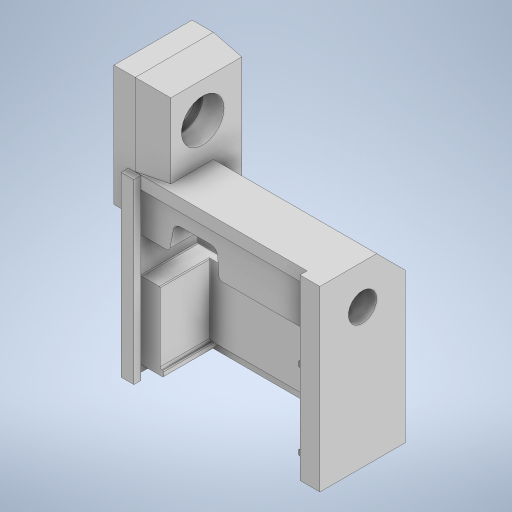
# Autodesk Inventor part: LimitSwitch Container
Saved by Autodesk Inventor 2023 (Build 270158000, 158)
## iProperties
Created: 2019-04-18
Part Number: LimitSwitch Container
Material: Generic
Document SubType Name: Modeling
Designer: Parker
Density: 1 g/cm^3
Appearance: Default
Author: Parker
Autodesk Inventor part; units mm, degrees
ref_plane "YZ Plane" through (0, 0, 0) normal (1, 0, 0) x (0, 1, 0)
sketch "Sketch1" plane through (0, 0, 0) normal (0, 0, 1) x (1, 0, 0)
  line L0 (-11.5, -20) -> (11.5, -20)
  line L1 (13.5, -18) -> (13.5, 18)
  line L2 (11.5, 20) -> (-11.5, 20)
  line L3 (-13.5, 18) -> (-13.5, -18)
  line L4 (-13.5, -20) -> (13.5, 20) construction
  line L5 (13.5, -20) -> (-13.5, 20) construction
  arc A0 (13.5, 18) -> (11.5, 20) centre (11.5, 18) ccw
  arc A1 (-11.5, 20) -> (-13.5, 18) centre (-11.5, 18) ccw
  arc A2 (-13.5, -18) -> (-11.5, -20) centre (-11.5, -18) ccw
  arc A3 (11.5, -20) -> (13.5, -18) centre (11.5, -18) ccw
  line L6 (12.7, 18) -> (12.7, -18)
  arc A4 (11.5, -19.2) -> (12.7, -18) centre (11.5, -18) ccw
  line L7 (11.5, -19.2) -> (-11.5, -19.2)
  arc A5 (-12.7, -18) -> (-11.5, -19.2) centre (-11.5, -18) ccw
  line L8 (-12.7, -18) -> (-12.7, 18)
  arc A6 (-11.5, 19.2) -> (-12.7, 18) centre (-11.5, 18) ccw
  line L9 (-11.5, 19.2) -> (11.5, 19.2)
  arc A7 (12.7, 18) -> (11.5, 19.2) centre (11.5, 18) ccw
  point P0 (0, 0)
  dimension "d0" = 27
  dimension "d1" = 40
  dimension "d2" = 2
  dimension "d3" = 0.8
  constraints: 20 end point, 16 point on circle, 8 centre point, 8 point on line, 8 tangent, 4 parallel, 3 equal radius, 2 midpoint, 2 perpendicular, 1 horizontal, 7 other
  measures "d0" distance of L4.end L5.end
  measures "d1" distance of L5.start L4.end
  measures "d2" radius of A0
  measures "d3" distance between parallel lines of L1 L6
extrude "Extrusion1" add sketch "Sketch1" along normal blind 10
sketch "Sketch2" plane through (13.5, -18, 0) normal (1, 0, 0) x (0, 0, -1)
  line L0 (-10, 0) -> (-10, 36) projected
  line L1 (0, 38) -> (-10, 38) projected
  point P0 (0, 18)
  point P1 (-5, 33.5)
  dimension "d6" = 5
  dimension "d7" = 4.5
  measures "d6" distance from line of L0 point (-5, 33.5)
  measures "d7" distance from line of L1 point (-5, 33.5)
ref_plane "Work Plane1" through (0, 0, 9) normal (0, 0, 1) x (1, 0, 0)
sketch "Sketch3" plane through (0, 0, 9) normal (0, 0, 1) x (1, 0, 0)
  arc A0 (-13.5, -18) -> (-11.5, -20) centre (-11.5, -18) ccw projected
  line L0 (-11.5, -20) -> (11.5, -20) projected
  arc A1 (11.5, -20) -> (13.5, -18) centre (11.5, -18) ccw projected
  line L1 (13.5, -18) -> (13.5, 18) projected
  arc A2 (13.5, 18) -> (11.5, 20) centre (11.5, 18) ccw projected
  line L2 (11.5, 20) -> (-11.5, 20) projected
  arc A3 (-11.5, 20) -> (-13.5, 18) centre (-11.5, 18) ccw projected
  line L3 (-13.5, 18) -> (-13.5, -18) projected
  line L4 (11.5, -19.2) -> (-11.5, -19.2) projected
  arc A4 (-12.7, -18) -> (-11.5, -19.2) centre (-11.5, -18) ccw projected
  line L5 (-12.7, -18) -> (-12.7, 18) projected
  arc A5 (-11.5, 19.2) -> (-12.7, 18) centre (-11.5, 18) ccw projected
  line L6 (-11.5, 19.2) -> (11.5, 19.2) projected
  arc A6 (12.7, 18) -> (11.5, 19.2) centre (11.5, 18) ccw projected
  line L7 (12.7, 18) -> (12.7, -18) projected
  arc A7 (11.5, -19.2) -> (12.7, -18) centre (11.5, -18) ccw projected
  line L8 (-12.7, 12.7) -> (12.7, 12.7)
  point P0 (0, 0)
  dimension "d16" = 6.5
  constraints: 2 end point, 2 point on line, 1 perpendicular
  measures "d16" distance between parallel lines of L8 L6
extrude "Extrusion2" add sketch "Sketch3" against normal blind 8 contours L8 L5 A5 L6 A6 L7
hole "Hole2" at (13.5, 15.5, 5) direction (-1, 0, 0) diameter 4 end through all
sketch "Sketch4" plane through (0, 0, 9) normal (0, 0, 1) x (1, 0, 0)
  line L0 (12.7, 18) -> (12.7, -18) projected
  line L1 (10, -2.3) -> (12.7, -2.3)
  line L2 (12.7, -2.3) -> (12.7, 7.7)
  line L3 (12.7, 7.7) -> (10, 7.7)
  line L4 (10, 7.7) -> (10, -2.3)
  line L5 (10, -2.3) -> (12.7, 7.7) construction
  line L6 (12.7, -2.3) -> (10, 7.7) construction
  line L7 (-10, -2.3) -> (-12.7, -2.3)
  line L8 (-12.7, -2.3) -> (-12.7, 7.7)
  line L9 (-12.7, 7.7) -> (-10, 7.7)
  line L10 (-10, 7.7) -> (-10, -2.3)
  line L11 (-10, -2.3) -> (-12.7, 7.7) construction
  line L12 (-12.7, -2.3) -> (-10, 7.7) construction
  arc A0 (-13.5, -18) -> (-11.5, -20) centre (-11.5, -18) ccw projected
  line L13 (-11.5, -20) -> (11.5, -20) projected
  arc A1 (11.5, -20) -> (13.5, -18) centre (11.5, -18) ccw projected
  line L14 (13.5, -18) -> (13.5, 18) projected
  arc A2 (13.5, 18) -> (11.5, 20) centre (11.5, 18) ccw projected
  line L15 (11.5, 20) -> (-11.5, 20) projected
  arc A3 (-11.5, 20) -> (-13.5, 18) centre (-11.5, 18) ccw projected
  line L16 (-13.5, 18) -> (-13.5, -18) projected
  line L17 (11.5, -19.2) -> (-11.5, -19.2) projected
  arc A4 (-12.7, -18) -> (-11.5, -19.2) centre (-11.5, -18) ccw projected
  line L18 (-12.7, -18) -> (-12.7, 18) projected
  arc A5 (-11.5, 19.2) -> (-12.7, 18) centre (-11.5, 18) ccw projected
  line L19 (-11.5, 19.2) -> (11.5, 19.2) projected
  arc A6 (12.7, 18) -> (11.5, 19.2) centre (11.5, 18) ccw projected
  line L20 (12.7, 18) -> (12.7, -18) projected
  arc A7 (11.5, -19.2) -> (12.7, -18) centre (11.5, -18) ccw projected
  line L21 (-12.7, 12.7) -> (12.7, 12.7) projected
  point P0 (0, 0)
  point P1 (11.35, 2.7)
  point P2 (-11.35, 2.7)
  dimension "d26" = 20
  dimension "d27" = 0
  dimension "d28" = 0
  dimension "d29" = 10
  dimension "d30" = 10
  dimension "d31" = 10
  dimension "d32" = 5
  constraints: 24 end point, 4 midpoint, 4 parallel, 2 horizontal, 2 perpendicular, 1 point on line
  measures "d26" distance between parallel lines of L4 L10
  measures "d27" distance between parallel lines of L18 L8
  measures "d28" distance from line of L1.start L7
  measures "d29" distance of L3.end L1.start
  measures "d30" distance of L9.end L7.start
  measures "d31" distance from line of point (0, 0) L4
  measures "d32" distance between parallel lines of L9 L21
extrude "Extrusion3" add sketch "Sketch4" against normal blind 8 contours L0 L1 L4 L3 | L9 L10 L7 L8
sketch "Sketch5" plane through (0, 0, 0) normal (0, 0, -1) x (-1, 0, 0)
  arc A0 (11.5, -20) -> (13.5, -18) centre (11.5, -18) ccw projected
  line L0 (13.5, 18) -> (13.5, -18) projected
  arc A1 (13.5, 18) -> (11.5, 20) centre (11.5, 18) ccw projected
  line L1 (-11.5, 20) -> (11.5, 20) projected
  arc A2 (-11.5, 20) -> (-13.5, 18) centre (-11.5, 18) ccw projected
  line L2 (-13.5, -18) -> (-13.5, 18) projected
  arc A3 (-13.5, -18) -> (-11.5, -20) centre (-11.5, -18) ccw projected
  line L3 (11.5, -20) -> (-11.5, -20) projected
  line L4 (-11.5, -19.2) -> (11.5, -19.2) projected
  arc A4 (-12.7, -18) -> (-11.5, -19.2) centre (-11.5, -18) ccw projected
  line L5 (-12.7, 18) -> (-12.7, -18) projected
  arc A5 (-11.5, 19.2) -> (-12.7, 18) centre (-11.5, 18) ccw projected
  line L6 (11.5, 19.2) -> (-11.5, 19.2) projected
  arc A6 (12.7, 18) -> (11.5, 19.2) centre (11.5, 18) ccw projected
  line L7 (12.7, -18) -> (12.7, 18) projected
  arc A7 (11.5, -19.2) -> (12.7, -18) centre (11.5, -18) ccw projected
  point P0 (0, 0)
extrude "Extrusion4" add sketch "Sketch5" against normal blind 1 contours A4 L5 A5 L6 A6 L7 A7 L4
sketch "Sketch6" plane through (0, 0, 9) normal (0, 0, 1) x (1, 0, 0)
  line L0 (-12.7, 12.7) -> (12.7, 12.7) projected
  line L1 (-11.7, 12.7) -> (-10.95, 16.45)
  line L2 (-10.95, 16.45) -> (-4.95, 16.45)
  line L3 (-4.95, 16.45) -> (-4.7, 12.7)
  line L4 (-12.7, -18) -> (-12.7, 18) projected
  point P0 (0, 0)
  dimension "d38" = 3.75
  dimension "d39" = 1
  dimension "d40" = 7
  dimension "d41" = 6
  dimension "d42" = 0.75
  constraints: 6 end point, 2 point on line, 1 horizontal
  measures "d38" distance between parallel lines of L0 L2
  measures "d39" distance from line of L4 L1.start
  measures "d40" distance of L1.start L3.end
  measures "d41" distance of L1.end L2.end
  measures "d42" horizontal distance of L1.start L1.end
extrude "Extrusion5" cut sketch "Sketch6" against normal blind 8
fillet "Fillet1" radius 0.5 2 edges at (-4.7, 12.7, 5) (-11.7, 12.7, 5)
fillet "Fillet2" radius 1 4 edges at (-10.95, 16.45, 7.88) (-10.95, 16.45, 2.12) (-4.95, 16.45, 7.88) (-4.95, 16.45, 2.12)
sketch "Sketch7" plane through (0, 0, 1) normal (0, 0, 1) x (1, 0, 0)
  line L0 (-10, 7.7) -> (-10, -2.3) projected
  line L1 (-10, 7.7) -> (2.5475, 7.7)
  line L2 (10, -2.3) -> (10, 7.7) projected
  line L3 (-10, -2.3) -> (10, -2.3)
  line L4 (10, -2.3) -> (10, 2.7)
  line L5 (10, 2.7) -> (3.2452, 2.7) construction
  line L6 (3.2452, 2.7) -> (2.5475, 7.7) construction
  spline S0 degree 2 poles (10, 2.7) (3.2452, 2.7) (2.5475, 7.7) knots 1 1 1 2 2 2
  point P0 (0, 0)
  constraints: 6 end point, 2 horizontal, 1 midpoint, 3 other
extrude "Extrusion6" add sketch "Sketch7" along normal blind 1
sketch "Sketch8" plane through (0, 0, 9) normal (0, 0, 1) x (1, 0, 0)
  line L0 (12.7, 7.7) -> (12.7, -2.3) projected
  line L1 (12.7, 7.7) -> (9.5, 7.7)
  line L2 (9.5, 7.7) -> (9.5, 8.5)
  line L3 (9.5, 8.5) -> (12.7, 8.5)
  line L4 (12.7, 8.5) -> (12.7, 7.7)
  line L5 (10, -2.3) -> (12.7, -2.3) projected
  line L6 (12.7, -2.3) -> (9.5, -2.3)
  line L7 (9.5, -2.3) -> (9.5, -3.1)
  line L8 (9.5, -3.1) -> (12.7, -3.1)
  line L9 (12.7, -3.1) -> (12.7, -2.3)
  line L10 (-12.7, -2.3) -> (-10, -2.3) projected
  line L11 (-12.7, -2.3) -> (-9.5, -2.3)
  line L12 (-9.5, -2.3) -> (-9.5, -3.1)
  line L13 (-9.5, -3.1) -> (-12.7, -3.1)
  line L14 (-12.7, -3.1) -> (-12.7, -2.3)
  line L15 (-10, -2.3) -> (-10, 7.7) projected
  line L16 (10, 7.7) -> (10, -2.3) projected
  point P0 (0, 0)
  dimension "d49" = 0.8
  dimension "d50" = 0.8
  dimension "d51" = 0.8
  dimension "d52" = 0.5
  dimension "d53" = 0.5
  dimension "d54" = 0.5
  constraints: 24 end point, 6 parallel, 3 horizontal, 3 perpendicular
  measures "d49" distance of L1.end L2.end
  measures "d50" distance of L6.end L7.end
  measures "d51" distance of L11.end L12.end
  measures "d52" distance between parallel lines of L12 L15
  measures "d53" distance between parallel lines of L16 L7
  measures "d54" distance between parallel lines of L16 L2
extrude "Extrusion7" add sketch "Sketch8" against normal blind 8 contours L1 L2 L3 L4 | L9 L8 L7 L6 L5 | L10 L11 L12 L13 L14
fillet "Fillet3" radius 0.25 3 edges at (10, 7.7, 5) (10, -2.3, 5.5) (-10, -2.3, 5.5)
fillet "Fillet4" radius 0.125 11 edges at (-9.5, -2.3, 5.5) (-9.5, -3.1, 5) (9.5, -3.1, 5) (9.5, -2.3, 5.5) (9.5, 7.7, 5) (9.5, 8.5, 5) (12.7, -3.1, 5) (12.7, 8.5, 5) (-12.7, 7.7, 5) (-10, 7.7, 5.5) (-12.7, -3.1, 5)
sketch "Sketch9" plane through (-11.5, -20, 0) normal (0, -1, 0) x (1, 0, 0)
  line L0 (0, 10) -> (23, 10) projected
  line L1 (11.5, 10) -> (11.5, 0) construction
  line L2 (10, 5) -> (13, 5)
  circle A0 centre (10, 5) radius 1
  circle A1 centre (13, 5) radius 1
  line L3 (10, 6) -> (13, 6)
  line L4 (13, 4) -> (10, 4)
  point P0 (11.5, 5)
  dimension "d59" = 3
  dimension "d60" = 1.5
  dimension "d61" = 2
  dimension "d62" = 2
  constraints: 8 end point, 4 point on circle, 2 centre point, 2 coincident, 2 midpoint, 2 tangent, 1 horizontal, 1 perpendicular
  measures "d59" distance of L2.start L2.end
  measures "d60" distance of point (11.5, 5) L2.end
  measures "d61" diameter of A0
  measures "d62" diameter of A1
extrude "Extrusion8" cut sketch "Sketch9" against normal up to next
sketch "Sketch11" plane through (0, 0, 10) normal (0, 0, 1) x (1, 0, 0)
  line L0 (13.5, -18) -> (13.5, 18) projected
  line L1 (13.5, -4.0701) -> (-15.3407, -4.0701)
  line L2 (-15.3407, -4.0701) -> (-15.3407, -24.8715)
  line L3 (-15.3407, -24.8715) -> (13.5, -24.8715)
  line L4 (13.5, -24.8715) -> (13.5, -4.0701)
  point P0 (0, 0)
  point P1 (13.5, -18)
  constraints: 8 end point, 2 parallel, 1 horizontal, 1 perpendicular, 1 point on line
extrude "Extrusion10" cut sketch "Sketch11" against normal through all
sketch "Sketch12" plane through (0, 0, 10) normal (0, 0, 1) x (1, 0, 0)
  line L0 (12.7, -4.0701) -> (13.5, -4.0701) projected
  line L1 (13.5, -4.0701) -> (13.5, 18) projected
  arc A0 (13.5, 18) -> (11.5, 20) centre (11.5, 18) ccw projected
  line L2 (11.5, 20) -> (-11.5, 20) projected
  arc A1 (-11.5, 20) -> (-13.5, 18) centre (-11.5, 18) ccw projected
  line L3 (-13.5, 18) -> (-13.5, -4.0701) projected
  line L4 (-13.5, -4.0701) -> (-12.7, -4.0701) projected
  line L5 (-12.7, -4.0701) -> (-12.7, 18) projected
  arc A2 (-11.5, 19.2) -> (-12.7, 18) centre (-11.5, 18) ccw projected
  line L6 (-11.5, 19.2) -> (11.5, 19.2) projected
  arc A3 (12.7, 18) -> (11.5, 19.2) centre (11.5, 18) ccw projected
  line L7 (12.7, 18) -> (12.7, -4.0701) projected
  line L8 (11.5, 20) -> (13.5, 20)
  arc A4 (13.5, 18) -> (11.5, 20) centre (11.5, 18) ccw projected
  line L9 (13.5, 20) -> (13.5, 18)
  line L10 (-13.5, 18) -> (-13.5, -4.0701) projected
  line L11 (-13.5, 18) -> (-13.5, 20)
  line L12 (-13.5, 20) -> (-11.5, 20)
  point P0 (0, 0)
  constraints: 8 end point, 2 point on line, 1 collinear, 1 horizontal, 1 perpendicular, 1 tangent
extrude "Extrusion11" add sketch "Sketch12" against normal up to surface (10 mm away) contours A0 L8 L9 | A1 L11 L12
sketch "Sketch13" plane through (-13.5, 20, 0) normal (-1, 0, 0) x (0, 0, 1)
  line L0 (0, -24.0701) -> (10, -24.0701) projected
  line L1 (10, 0) -> (10, -24.0701) projected
  line L2 (0, -24.0701) -> (0, 0) projected
  circle A0 centre (5, -4.5) radius 2 projected
  line L3 (0, 0) -> (0, -24.0701) projected
  line L4 (0, -12.9) -> (10, -12.9)
  line L5 (10, -12.9) -> (10, 12.5)
  line L6 (10, 12.5) -> (0, 12.5)
  line L7 (0, 12.5) -> (0, -12.9)
  line L8 (-1, -13.4) -> (-20.5, -13.4) projected
  line L9 (-59, 12.5) -> (-1, 12.5) projected
  line L10 (10, 0) -> (0, 0) projected
  point P0 (0, -20)
  point P1 (0, -12.9)
  point P2 (10, -12.9)
  dimension "d73" = 0.5
  dimension "d74" = 0
  constraints: 8 end point, 2 parallel, 1 horizontal, 1 perpendicular, 1 point on line
  measures "d73" distance between parallel lines of L8 L4
  measures "d74" distance between parallel lines of L9 L6
ref_plane "Work Plane2" through (-14.5, 15.5, -59) normal (1, 0, 0) x (0, 1, 0)
extrude "Extrusion12" add sketch "Sketch13" along normal up to surface (1 mm away) contours L2 L10 L1 L4 | L7 L6 L5 L10 | A0
sketch "Sketch14" plane through (-13.5, 20, 0) normal (1, 0, 0) x (0, 0, -1)
  line L0 (-10, 0) -> (0, 0) projected
  line L1 (0, 12.5) -> (0, 0) projected
  line L2 (-10, 12.5) -> (0, 12.5) projected
  line L3 (-10, 0) -> (-10, 12.5) projected
  point P0 (0, -20)
extrude "Extrusion13" add sketch "Sketch14" along normal blind 5
move faces "Move1" translate (0, 1, 0) faces at (6.1667, 20, 3.3333)
move faces "Move2" translate (0, 0, -1) faces at (4.5, 8.01, 0)
move faces "Move3" translate (1, 0, 0) faces at (13.5, 1.7915, 4.5863)
sketch "Sketch15" plane through (-8.5, 20, 0) normal (1, 0, 0) x (0, 0, -1)
  line L0 (1, 1) -> (1, 12.5) projected
  line L1 (-10, 1) -> (1, 1) projected
  point P0 (0, -20)
  point P1 (-4.5, 6.5)
  dimension "d88" = 5.5
  dimension "d89" = 5.5
  measures "d88" distance from line of L0 point (-4.5, 6.5)
  measures "d89" distance from line of L1 point (-4.5, 6.5)
hole "Hole3" at (-8.5, 26.5, 4.5) direction (-1, 0, 0) diameter 3.6 end through all counterbore diameter 6 counterbore depth 3
chamfer "Chamfer1" distance 1 distance2 4 1 edges at (-8.5, 32.5, 4.5) measured on face at (-8.5, 32, 4.5)
chamfer "Chamfer2" distance 1 distance2 4 1 edges at (-8.5, 26.25, 10) measured on face at (-8.5, 26.25, 9.5)
sketch "Sketch16" plane through (0, 0, 10) normal (0, 0, 1) x (1, 0, 0)
  line L0 (-13.5, -4.0701) -> (-13.5, 7.1) projected
  line L1 (-13.5, -4.0701) -> (-11.7, -4.0701)
  line L2 (-11.7, -4.0701) -> (-11.7, 20.9299)
  line L3 (-11.7, 20.9299) -> (-13.5, 20.9299)
  line L4 (-13.5, 20.9299) -> (-13.5, -4.0701)
  line L5 (14.5, -4.0701) -> (-13.5, -4.0701) projected
  line L6 (-8.5, 21) -> (14.5, 21) projected
  line L7 (14.5, -4.0701) -> (11.7, -4.0701)
  line L8 (11.7, -4.0701) -> (11.7, 21)
  line L9 (11.7, 21) -> (14.5, 21)
  line L10 (14.5, 21) -> (14.5, -4.0701)
  line L11 (12.7, 18) -> (12.7, -4.0701) projected
  line L12 (-12.7, -4.0701) -> (-12.7, 18) projected
  point P0 (0, 0)
  dimension "d103" = 25
  dimension "d105" = 1
  dimension "d106" = 1
  constraints: 16 end point, 4 parallel, 2 horizontal, 2 perpendicular, 1 point on line
  measures "d103" distance of L2.end L1.end
  measures "d105" distance between parallel lines of L11 L8
  measures "d106" distance between parallel lines of L12 L2
extrude "Extrusion14" add sketch "Sketch16" along normal blind 1
sketch "Sketch17" plane through (-14.5, 7.1, 10) normal (-1, 0, 0) x (0, 0, 1)
  circle A0 centre (-5.5, 19.4) radius 1.8 projected
  line L0 (0, 25.4) -> (-11, 25.4) projected
  line L1 (-11, 25.4) -> (-11, 0) projected
  line L2 (-11, 0) -> (0, 0) projected
  line L3 (0, 0) -> (0, 25.4) projected
  line L4 (-7, 8.4) -> (-11, 8.4) projected
  line L5 (-11, 8.4) -> (0, 8.4)
  point P0 (-10, -7.1)
  constraints: 2 end point, 2 point on line
extrude "Extrusion15" add sketch "Sketch17" along normal blind 1 contours L3 L5 L4 L1 L0
chamfer "Chamfer3" distance 4 angle 45 1 edges at (3, 21, -1)
sketch "Sketch18" plane through (14.5, -4.0701, 11) normal (1, 0, 0) x (0, 0, -1)
  circle A0 centre (6, 19.5701) radius 2 projected
  point P0 (11, 4.0701)
extrude "Extrusion16" cut sketch "Sketch18" against normal through all
move faces "Move4" translate (3, 0, 0) faces at (-7.3004, 16.45, 2.4934) (-7.3004, 16.45, 8.2533) (-11.3351, 14.5245, 8.2943) (-10.279, 16.4389, 8.2576) (-10.279, 16.4389, 1.7424) (-11.7378, 12.866, 6.3333) (-4.5605, 12.8229, 6.3333) (-4.8179, 14.4682, 1.7193) (-5.7732, 16.4437, 1.7453) (-5.7732, 16.4437, 8.2547)
body "Solid1"
